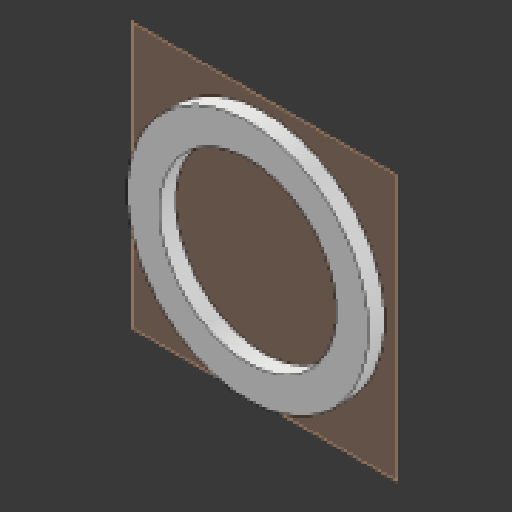
# Autodesk Inventor part: Ring
Saved by Autodesk Inventor 2023 (Build 270158000, 158)
## iProperties
Created: 2023-03-16
Part Number: Ring
Material: Generic
Document SubType Name: Modeling
Designer: alber
Density: 1 g/cm^3
Appearance: Default
Author: alber
Autodesk Inventor part; units mm, degrees
ref_plane "YZ Plane" through (0, 0, 0) normal (1, 0, 0) x (0, 1, 0)
ref_plane "XZ Plane" through (0, 0, 0) normal (0, 1, 0) x (-1, 0, 0)
ref_plane "XY Plane" through (0, 0, 0) normal (0, 0, 1) x (1, 0, 0)
ref_plane "Work Plane1" through (18.0089, -8.7705, -24.5078) normal (0, 0, 1) x (1, 0, 0)
sketch "Sketch1" plane through (18.0089, -8.7705, -24.5078) normal (0, 0, 1) x (1, 0, 0)
  circle A0 centre (0, 0) radius 30 projected
  circle A1 centre (0, 0) radius 30
  circle A2 centre (0, 0) radius 22
  point P0 (-18.0089, 8.7705)
  dimension "d0" = 60
  dimension "d1" = 8
  constraints: 2 centre point, 1 coincident
  measures "d0" diameter of A1
  measures "d1" radial gap between concentric circles of A0 A2
extrude "Extrusion1" add sketch "Sketch1" along normal blind 4
body "Solid1"
